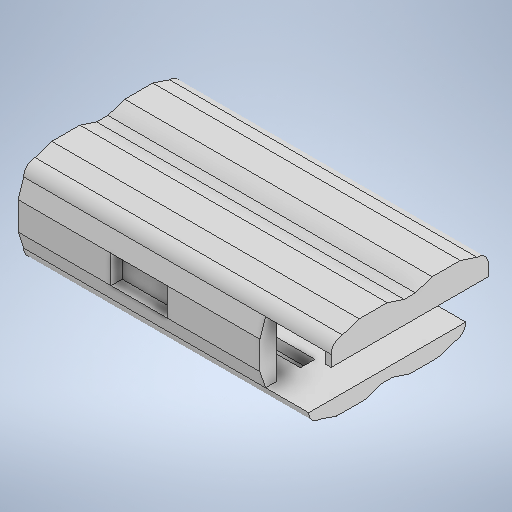
# Autodesk Inventor part: magasin
Saved by Autodesk Inventor 2025 (Build 290162000, 162)
## iProperties
Created: 2026-07-08
Part Number: magasin
Material: Типовые
Document SubType Name: Modeling
Designer: garin
Density: 1 g/cm^3
Appearance: По умолчанию
Author: garin
Autodesk Inventor part; units mm, degrees
ref_plane "YZ Plane" through (0, 0, 0) normal (1, 0, 0) x (0, 1, 0)
ref_plane "XZ Plane" through (0, 0, 0) normal (0, 1, 0) x (-1, 0, 0)
ref_plane "XY Plane" through (0, 0, 0) normal (0, 0, 1) x (1, 0, 0)
sketch "Эскиз1" plane through (0, 0, 0) normal (1, 0, 0) x (0, 1, 0)
  line L0 (11, 12) -> (0, 12)
  line L1 (0, 12) -> (0, 1)
  line L2 (0, 1) -> (11, 1)
  line L3 (11, 1) -> (11, 12)
  line L4 (0, 0) -> (0, 1) construction
  line L5 (0, 0) -> (15, 0) construction
  line L6 (11, -12) -> (0, -12)
  line L7 (0, -12) -> (0, -1)
  line L8 (0, -1) -> (11, -1)
  line L9 (11, -1) -> (11, -12)
  line L10 (11, 12) -> (13, 12) construction
  line L11 (13, 12) -> (13, 14) construction
  line L12 (13, 14) -> (11, 14) construction
  line L13 (11, 14) -> (11, 12)
  line L14 (13, 14) -> (1, 14)
  line L15 (1, 14) -> (1, -14)
  line L16 (1, -14) -> (13, -14)
  line L17 (13, -14) -> (13, 14)
  line L18 (1, 14) -> (-2, 14)
  line L19 (-2, 14) -> (-2, -14)
  line L20 (-2, -14) -> (1, -14)
  line L21 (1, -14) -> (1, 14)
  line L22 (13, 14) -> (9, 14)
  line L23 (9, 14) -> (9, -14)
  line L24 (9, -14) -> (13, -14)
  line L25 (13, -14) -> (13, 14)
  line L26 (11, -12) -> (11, -14)
  line L27 (11, 1) -> (8, 1) construction
  line L28 (8, 1) -> (8, 4) construction
  line L29 (8, 4) -> (11, 4) construction
  line L30 (11, 4) -> (11, 1) construction
  line L31 (8, 4) -> (3, 4)
  line L32 (3, 4) -> (3, 9)
  line L33 (3, 9) -> (8, 9)
  line L34 (8, 9) -> (8, 4)
  line L35 (8, -4) -> (3, -4)
  line L36 (3, -4) -> (3, -9)
  line L37 (3, -9) -> (8, -9)
  line L38 (8, -9) -> (8, -4)
  line L39 (0, 12) -> (0, 14)
  line L40 (0, -1) -> (0, 1)
  line L41 (0, -12) -> (0, -14)
  line L42 (0, 12) -> (-2, 12) construction
  line L43 (-2, 12) -> (-3, 12) construction
  line L44 (-3, 12) -> (-3, 9) construction
  line L45 (-3, 9) -> (-2, 9) construction
  line L46 (-2, 9) -> (-2, 12) construction
  line L47 (0, 1) -> (-2, 1) construction
  line L48 (-2, 1) -> (-3, 1) construction
  line L49 (-3, 1) -> (-3, 4) construction
  line L50 (-3, 4) -> (-2, 4) construction
  line L51 (-2, 4) -> (-2, 1) construction
  line L52 (-2, 12) -> (-3, 9)
  line L53 (-3, 9) -> (-3, 4)
  line L54 (-3, 4) -> (-2, 1)
  line L55 (-2, 9) -> (-2.2, 9) construction
  line L56 (-2.2, 9) -> (-2.2, 4) construction
  line L57 (-2.2, 4) -> (-2, 4) construction
  line L58 (-2, 4) -> (-2, 9) construction
  line L59 (-2.2, 9) -> (-1, 9)
  line L60 (-1, 9) -> (-1, 4)
  line L61 (-1, 4) -> (-2.2, 4)
  line L62 (-2.2, 4) -> (-2.2, 9)
  line L63 (-1, 9) -> (-1, 7.8) construction
  line L64 (-1, 7.8) -> (0, 7.8)
  line L65 (0, 7.8) -> (0, 5.2)
  line L66 (0, 5.2) -> (-1, 5.2)
  line L67 (-1, 5.2) -> (-1, 7.8)
  line L68 (-2, -12) -> (-3, -9)
  line L69 (-3, -9) -> (-3, -4)
  line L70 (-3, -4) -> (-2, -1)
  line L71 (-2.2, -9) -> (-1, -9)
  line L72 (-1, -9) -> (-1, -4)
  line L73 (-1, -4) -> (-2.2, -4)
  line L74 (-2.2, -4) -> (-2.2, -9)
  line L75 (-1, -7.8) -> (0, -7.8)
  line L76 (0, -5.2) -> (-1, -5.2)
  line L77 (5.5, 4) -> (5.5, -4) construction
  line L78 (13, 12) -> (14, 9)
  line L79 (14, 9) -> (14, 4)
  line L80 (14, 4) -> (13, 1)
  line L81 (13.2, 9) -> (12, 9)
  line L82 (12, 9) -> (12, 4)
  line L83 (12, 4) -> (13.2, 4)
  line L84 (13.2, 4) -> (13.2, 9)
  line L85 (12, 7.8) -> (11, 7.8)
  line L86 (11, 5.2) -> (12, 5.2)
  line L87 (14, -9) -> (14, -4)
  line L88 (14, -4) -> (13, -1)
  line L89 (12, -4) -> (13.2, -4)
  line L90 (13.2, -4) -> (13.2, -9)
  line L91 (13.2, -9) -> (12, -9)
  line L92 (12, -9) -> (12, -4)
  line L93 (12, -7.8) -> (11, -7.8)
  line L94 (11, -5.2) -> (12, -5.2)
  line L95 (13, -12) -> (14, -9)
  line L96 (-1, 7.8) -> (-2, 7.8)
  line L97 (-2, 7.8) -> (-2, 5.2)
  line L98 (-2, 5.2) -> (-1, 5.2)
  line L99 (-1, 5.2) -> (-1, 7.8)
  line L100 (-1, -5.2) -> (-1, -7.8)
  line L101 (-1, -7.8) -> (-2, -7.8)
  line L102 (-2, -7.8) -> (-2, -5.2)
  line L103 (-2, -5.2) -> (-1, -5.2)
  line L104 (-1, -5.2) -> (-1, -7.8)
  line L105 (12, 5.2) -> (12, 7.8)
  line L106 (12, 7.8) -> (13, 7.8)
  line L107 (13, 7.8) -> (13, 5.2)
  line L108 (13, 5.2) -> (12, 5.2)
  line L109 (12, 5.2) -> (12, 7.8)
  line L110 (12, -7.8) -> (13, -7.8)
  line L111 (13, -7.8) -> (13, -5.2)
  line L112 (13, -5.2) -> (12, -5.2)
  line L113 (12, -5.2) -> (12, -7.8)
  line L114 (12, -5.2) -> (12, -7.8)
  line L115 (0, 14) -> (3, 14) construction
  line L116 (3, 14) -> (3, 15) construction
  line L117 (3, 15) -> (0, 15) construction
  line L118 (0, 15) -> (0, 14) construction
  line L119 (11, 14) -> (8, 14) construction
  line L120 (8, 14) -> (8, 15) construction
  line L121 (8, 15) -> (11, 15) construction
  line L122 (11, 15) -> (11, 14) construction
  line L123 (11, 14) -> (8, 15)
  line L124 (8, 15) -> (3, 15)
  line L125 (0, 14) -> (3, 15)
  line L126 (0, -14) -> (3, -14) construction
  line L127 (3, -14) -> (3, -15) construction
  line L128 (3, -15) -> (0, -15) construction
  line L129 (0, -15) -> (0, -14) construction
  line L130 (11, -14) -> (8, -14) construction
  line L131 (8, -14) -> (8, -15) construction
  line L132 (8, -15) -> (11, -15) construction
  line L133 (11, -15) -> (11, -14) construction
  line L134 (11, -14) -> (8, -15)
  line L135 (8, -15) -> (3, -15)
  line L136 (0, -14) -> (3, -15)
  point P0 (9, 1)
  point P1 (9, -1)
  point P2 (11, -14)
  point P3 (0, -12)
  point P4 (0, -1)
  point P5 (0, 1)
  point P6 (0, 12)
  point P7 (1, -1)
  point P8 (1, -12)
  dimension "d0" = 11
  dimension "d1" = 11
  dimension "d2" = 1
  dimension "d3" = 15
  dimension "d4" = 2
  dimension "d5" = 2
  dimension "d6" = 12
  dimension "d7" = 28
  dimension "d8" = 3
  dimension "d9" = 28
  dimension "d10" = 4
  dimension "d11" = 3
  dimension "d12" = 3
  dimension "d13" = 5
  dimension "d14" = 5
  dimension "d44" = 1
  dimension "d45" = 3
  dimension "d46" = 1
  dimension "d47" = 3
  dimension "d48" = 0.2
  dimension "d49" = 1.2
  dimension "d50" = 5
  dimension "d51" = 1.2
  dimension "d52" = 1
  dimension "d53" = 2.6
  dimension "d60" = 1
  dimension "d61" = 3
  dimension "d62" = 1
  dimension "d63" = 3
  dimension "d64" = 1
  constraints: 274 end point, 62 symmetric about line, 31 equal length, 19 perpendicular, 16 horizontal, 12 point on line, 3 midpoint, 1 vertical
  measures "d0" distance of L1.end L2.end
  measures "d1" distance of L1.end L0.end
  measures "d2" distance of L4.start L1.end
  measures "d3" distance of L4.start L5.end
  measures "d4" distance of L12.end L11.end
  measures "d5" distance of L11.end L10.end
  measures "d6" distance of L16.end L15.end
  measures "d7" distance of L15.end L14.end
  measures "d8" distance of L20.end L19.end
  measures "d9" distance of L19.end L18.end
  measures "d10" distance of L24.end L23.end
  measures "d11" distance of L28.end L29.end
  measures "d12" distance of L27.end L28.end
  measures "d13" distance of L32.end L33.end
  measures "d14" distance of L31.end L32.end
  measures "d44" distance of L45.end L44.end
  measures "d45" distance of L44.end L43.end
  measures "d46" distance of L49.end L50.end
  measures "d47" distance of L48.end L49.end
  measures "d48" distance of L57.end L56.end
  measures "d49" distance of L60.end L61.end
  measures "d50" distance of L59.end L60.end
  measures "d51" distance of L59.end L63.end
  measures "d52" distance of L65.end L66.end
  measures "d53" distance of L64.end L65.end
  measures "d60" distance of L98.end L97.end
  measures "d61" distance of L117.end L116.end
  measures "d62" distance of L116.end L115.end
  measures "d63" distance of L120.end L121.end
  measures "d64" distance of L119.end L120.end
extrude "Выдавливание1" add sketch "Эскиз1" along normal blind 0.8 contours L3 L2 L23 L0 | L13 L14 L17 L81 L82 L85 L3 | L0 L23 L14 L13 | L23 L2 L15 L0 | L0 L15 L14 L23 | L85 L82 L86 L3 | L15 L2 L1 L0 | L0 L39 L18 L15 | L23 L8 L15 L2 | L2 L3 L86 L82 L83 L17 L89 L92 L94 L9 L8 L23 | L106 L17 L108 L82 | L82 L81 L17 L106 | L1 L64 L60 L59 L19 L18 L39 | L15 L8 L40 L2 | L23 L6 L15 L8 | L8 L9 L6 L23 | L108 L17 L83 L82 | L1 L66 L60 L64 | L40 L7 L76 L72 L73 L19 L61 L60 L66 L1 | L15 L6 L7 L8 | L23 L16 L15 L6 | L6 L26 L16 L23 | L96 L19 L59 L60 | L60 L98 L19 L96 | L15 L20 L41 L6 | L94 L92 L93 L9 | L9 L93 L92 L91 L17 L16 L26 | L60 L61 L19 L98 | L7 L75 L72 L76 | L41 L20 L19 L71 L72 L75 L7 | L112 L17 L110 L92 | L92 L89 L17 L112 | L103 L19 L73 L72 | L72 L101 L19 L103 | L110 L17 L91 L92 | L72 L71 L19 L101
extrude "Выдавливание2" add sketch "Эскиз1" along normal blind 43.1 contours L13 L14 L17 L81 L82 L85 L3 | L0 L23 L14 L13 | L0 L15 L14 L23 | L85 L82 L86 L3 | L0 L39 L18 L15 | L23 L8 L15 L2 | L2 L3 L86 L82 L83 L17 L89 L92 L94 L9 L8 L23 | L106 L17 L108 L82 | L82 L81 L17 L106 | L1 L64 L60 L59 L19 L18 L39 | L15 L8 L40 L2 | L108 L17 L83 L82 | L1 L66 L60 L64 | L40 L7 L76 L72 L73 L19 L61 L60 L66 L1 | L23 L16 L15 L6 | L6 L26 L16 L23 | L96 L19 L59 L60 | L60 L98 L19 L96 | L15 L20 L41 L6 | L94 L92 L93 L9 | L9 L93 L92 L91 L17 L16 L26 | L60 L61 L19 L98 | L7 L75 L72 L76 | L41 L20 L19 L71 L72 L75 L7 | L112 L17 L110 L92 | L92 L89 L17 L112 | L103 L19 L73 L72 | L72 L101 L19 L103 | L110 L17 L91 L92 | L72 L71 L19 L101
extrude "Выдавливание3" add sketch "Эскиз1" along normal blind 10.7 from surface at 43.1 contours L13 L14 L17 L81 L82 L85 L3 | L85 L82 L86 L3 | L2 L3 L86 L82 L83 L17 L89 L92 L94 L9 L8 L23 | L106 L17 L108 L82 | L82 L81 L17 L106 | L108 L17 L83 L82 | L94 L92 L93 L9 | L9 L93 L92 L91 L17 L16 L26 | L112 L17 L110 L92 | L92 L89 L17 L112 | L110 L17 L91 L92
extrude "Выдавливание4" add sketch "Эскиз1" along normal blind 1 from surface at 53.8 contours L3 L2 L23 L0 | L13 L14 L17 L81 L82 L85 L3 | L0 L23 L14 L13 | L85 L82 L86 L3 | L2 L3 L86 L82 L83 L17 L89 L92 L94 L9 L8 L23 | L106 L17 L108 L82 | L82 L81 L17 L106 | L8 L9 L6 L23 | L108 L17 L83 L82 | L6 L26 L16 L23 | L94 L92 L93 L9 | L9 L93 L92 L91 L17 L16 L26 | L112 L17 L110 L92 | L92 L89 L17 L112 | L110 L17 L91 L92
sketch "Эскиз2" plane through (0, 13, 14) normal (0, 1, 0) x (1, 0, 0)
  line L0 (0, 28) -> (43.1, 28) construction
  line L1 (0, 0) -> (10.8, 0) construction
  line L2 (10.8, 0) -> (10.8, 28) construction
  line L3 (10.8, 28) -> (0, 28) construction
  line L4 (0, 28) -> (0, 0) construction
  line L5 (10.8, 14) -> (54.8, 14) construction
  line L6 (54.8, 28) -> (54.8, 0) construction
  line L7 (10.8, 14) -> (54.8, 14) construction
  line L8 (54.8, 14) -> (54.8, 15) construction
  line L9 (54.8, 15) -> (10.8, 15) construction
  line L10 (10.8, 15) -> (10.8, 14) construction
  line L11 (10.8, 14) -> (54.8, 14) construction
  line L12 (54.8, 14) -> (54.8, 13) construction
  line L13 (54.8, 13) -> (10.8, 13) construction
  line L14 (10.8, 13) -> (10.8, 14) construction
  line L15 (32.8, 15) -> (32.8, 28) construction
  line L16 (32.8, 21.5) -> (10.8, 21.5) construction
  line L17 (32.8, 21.5) -> (54.8, 21.5) construction
  line L18 (10.8, 21.5) -> (21.8, 21.5) construction
  line L19 (21.8, 21.5) -> (21.8, 28) construction
  line L20 (21.8, 28) -> (10.8, 28) construction
  line L21 (10.8, 28) -> (10.8, 21.5) construction
  line L22 (21.8, 21.5) -> (32.8, 21.5) construction
  line L23 (32.8, 21.5) -> (32.8, 28) construction
  line L24 (32.8, 28) -> (21.8, 28) construction
  line L25 (21.8, 28) -> (21.8, 21.5) construction
  line L26 (32.8, 21.5) -> (43.8, 21.5) construction
  line L27 (43.8, 21.5) -> (43.8, 28) construction
  line L28 (43.8, 28) -> (32.8, 28) construction
  line L29 (32.8, 28) -> (32.8, 21.5) construction
  line L30 (43.8, 21.5) -> (54.8, 21.5) construction
  line L31 (54.8, 21.5) -> (54.8, 28) construction
  line L32 (54.8, 28) -> (43.8, 28) construction
  line L33 (43.8, 28) -> (43.8, 21.5) construction
  line L34 (49.3, 21.5) -> (49.3, 28) construction
  line L35 (38.3, 21.5) -> (38.3, 28) construction
  line L36 (27.3, 21.5) -> (27.3, 28) construction
  line L37 (16.3, 21.5) -> (16.3, 28) construction
  circle A0 centre (16.3, 21.5) radius 2
  circle A1 centre (27.3, 21.5) radius 2
  circle A2 centre (38.3, 21.5) radius 2
  circle A3 centre (49.3, 21.5) radius 2
  circle A4 centre (16.3, 6.5) radius 2
  circle A5 centre (27.3, 6.5) radius 2
  circle A6 centre (38.3, 6.5) radius 2
  circle A7 centre (49.3, 6.5) radius 2
  line L38 (0, 28) -> (4, 28) construction
  line L39 (4, 28) -> (4, 23) construction
  line L40 (4, 23) -> (0, 23) construction
  line L41 (0, 23) -> (0, 28) construction
  line L42 (4, 23) -> (7, 23)
  line L43 (7, 23) -> (7, 6)
  line L44 (7, 6) -> (4, 6)
  line L45 (4, 6) -> (4, 23)
  point P0 (0, 14)
  point P1 (54.7, 26)
  dimension "d23" = 10.8
  dimension "d27" = 1
  dimension "d28" = 1
  dimension "d29" = 11
  dimension "d30" = 11
  dimension "d31" = 11
  dimension "d32" = 11
  dimension "d33" = 4
  dimension "d34" = 4
  dimension "d35" = 4
  dimension "d36" = 4
  dimension "d39" = 4
  dimension "d40" = 5
  dimension "d41" = 3
  dimension "d42" = 17
  constraints: 88 end point, 18 parallel, 12 midpoint, 10 perpendicular, 9 horizontal, 8 centre point, 6 point on line, 4 coincident, 4 symmetric about line, 1 vertical, 10 other
  measures "d23" distance of L3.end L2.end
  measures "d27" distance of L8.end L7.end
  measures "d28" distance of L11.end L12.end
  measures "d29" distance of L20.end L19.end
  measures "d30" distance of L24.end L23.end
  measures "d31" distance of L28.end L27.end
  measures "d32" distance of L32.end L31.end
  measures "d33" diameter of A0
  measures "d34" diameter of A1
  measures "d35" diameter of A2
  measures "d36" diameter of A3
  measures "d39" distance of L39.end L40.end
  measures "d40" distance of L38.end L39.end
  measures "d41" distance of L43.end L44.end
  measures "d42" distance of L42.end L43.end
extrude "Выдавливание5" add sketch "Эскиз1" along normal blind 7.7 from surface at 43.1 contours L1 L64 L60 L59 L19 L18 L39 | L1 L66 L60 L64 | L40 L7 L76 L72 L73 L19 L61 L60 L66 L1 | L96 L19 L59 L60 | L60 L98 L19 L96 | L60 L61 L19 L98 | L7 L75 L72 L76 | L41 L20 L19 L71 L72 L75 L7 | L103 L19 L73 L72 | L72 L101 L19 L103 | L72 L71 L19 L101
extrude "Выдавливание7" add sketch "Эскиз1" along normal blind 54.8 contours L17 L81 L84 L83 | L78 L79 L80 L17 L83 L84 L81 | L17 L89 L90 L91 | L88 L87 L95 L17 L91 L90 L89
extrude "Выдавливание8" add sketch "Эскиз1" along normal blind 50.8 contours L19 L61 L62 L59 | L19 L59 L62 L61 L54 L53 L52 | L19 L71 L74 L73 | L73 L74 L71 L19 L68 L69 L70
extrude "Выдавливание9" cut sketch "Эскиз1" along normal blind 42.3 from surface at 0.8 contours L85 L82 L86 L3 | L106 L17 L108 L82 | L1 L66 L60 L64 | L60 L98 L19 L96 | L94 L92 L93 L9 | L7 L75 L72 L76 | L112 L17 L110 L92 | L72 L101 L19 L103
extrude "Выдавливание10" add sketch "Эскиз1" along normal blind 43.1 contours L14 L18 L125 L124 L123 | L16 L134 L135 L136 L20
sketch "Эскиз5" plane through (0, 3, -15) normal (0, 0, -1) x (-1, 0, 0)
  line L0 (0, 0) -> (-0.8, 0) projected
  line L1 (0, 5) -> (-43.1, 5) projected
  line L2 (0, 0) -> (-43.1, 0)
  line L3 (-43.1, 0) -> (-43.1, 5)
  line L4 (-43.1, 5) -> (0, 5)
  line L5 (0, 5) -> (0, 0)
  line L6 (-26.55, 5) -> (-16.55, 5)
  line L7 (-16.55, 5) -> (-16.55, 0)
  line L8 (-16.55, 0) -> (-26.55, 0)
  line L9 (-26.55, 0) -> (-26.55, 5)
  point P0 (0, -3)
  point P1 (-21.55, 5)
  dimension "d67" = 10
  dimension "d68" = 5
  constraints: 16 end point, 4 parallel, 2 horizontal, 2 midpoint, 2 perpendicular
  measures "d67" distance of L7.end L8.end
  measures "d68" distance of L6.end L7.end
extrude "Выдавливание11" cut sketch "Эскиз5" against normal blind 2 contours L2 L9 L1 L7
extrude "Выдавливание12" cut sketch "Эскиз5" along normal blind 2 from surface at -30 contours L2 L9 L1 L7
fillet "Сопряжение2" radius 2 14 edges at (27.4, 13, -14) (25.4, -2, -14) (27.4, 13, 14) (25.4, -2, 14) (0.4, 3, -9) (0.4, 3, 4) (0.4, 8, 4) (0.4, 8, -9) (0.4, 8, 9) (0.4, 3, 9) (0.4, 3, -4) (0.4, 8, -4) (43.1, 9, 0) (43.1, 0, 0)
